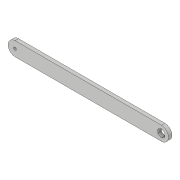
# Autodesk Inventor part: Piv arm
Saved by Autodesk Inventor 2018 (Build 220112000, 112)
## iProperties
Created: 2017-12-19
Part Number: Piv arm
Material: Generic
Document SubType Name: Modeling
Designer: dsayers
Density: 1 g/cm^3
Appearance: Default
Author: dsayers
Autodesk Inventor part; units mm, degrees
ref_plane "YZ Plane" through (0, 0, 0) normal (1, 0, 0) x (0, 1, 0)
ref_plane "XZ Plane" through (0, 0, 0) normal (0, 1, 0) x (-1, 0, 0)
ref_plane "XY Plane" through (0, 0, 0) normal (0, 0, 1) x (1, 0, 0)
sketch "Sketch1" plane through (0, 0, 0) normal (0, 0, 1) x (1, 0, 0)
  line L0 (0, 7.3323) -> (6.35, 3.6662)
  line L1 (6.35, 3.6662) -> (6.35, -3.6662)
  line L2 (6.35, -3.6662) -> (0, -7.3323)
  line L3 (0, -7.3323) -> (-6.35, -3.6662)
  line L4 (-6.35, -3.6662) -> (-6.35, 3.6662)
  line L5 (-6.35, 3.6662) -> (0, 7.3323)
  circle A0 centre (-266.7, 0) radius 2.54
  line L6 (-266.7, 0) -> (0, 0) construction
  line L7 (-266.7, -12.7) -> (0, -12.7)
  line L8 (0, 12.7) -> (-266.7, 12.7)
  arc A1 (-266.7, 12.7) -> (-266.7, -12.7) centre (-266.7, 0) ccw
  arc A2 (0, -12.7) -> (0, 12.7) centre (0, 0) ccw
  point P0 (-133.35, 0)
  dimension "d0" = 12.7
  dimension "d1" = 5.08
  dimension "d2" = 266.7
  dimension "d3" = 25.4
  constraints: 20 end point, 4 point on circle, 4 tangent, 3 centre point, 1 coincident, 1 horizontal, 1 midpoint, 1 parallel, 13 other
  measures "d0" distance between parallel lines of L3 L0
  measures "d1" diameter of A0
  measures "d2" distance of point (0, 0) L6.start
  measures "d3" distance between parallel lines of L8 L7
extrude "Extrusion1" add sketch "Sketch1" along normal blind 6.35
body "Solid1"
